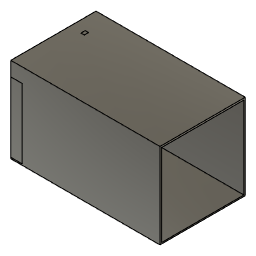
ufo-hanger-with-door (Autodesk Fusion 360 design; units mm, degrees)
Autodesk Fusion 360 part; units mm, degrees
sketch "Sketch1" plane through (0, 0, 0) normal (0, 1, 0) x (1, 0, 0)
  line L0 (0, -120) -> (101.6, -120)
  line L1 (101.6, -120) -> (101.6, 57.8)
  line L2 (101.6, 57.8) -> (0, 57.8)
  line L3 (0, 57.8) -> (0, -120)
  dimension "d1" = 101.6
  dimension "d2" = 177.8
  constraint horizontal L0
  constraint vertical L1
  constraint horizontal L2
  constraint vertical L3
  measures "d1" distance of L0.start L0.end
  measures "d2" distance of L0.start L2.end
extrude "Extrude1" add sketch "Sketch1" along normal blind 101.6 makes body 1
move_body "Move1" bodies 1 to x (0, 0, 1) y (0, 1, 0) z (-1, 0, 0) at (53.5039, 0, 53.5039)
sketch "Sketch2" plane through (-66.4961, 0, 0) normal (-1, 0, 0) x (0, -1, 0)
  line L0 (0, 53.5039) -> (0, 155.1039)
  line L1 (0, 155.1039) -> (-101.6, 155.1039)
  line L2 (-101.6, 155.1039) -> (-101.6, 53.5039)
  line L3 (-101.6, 53.5039) -> (0, 53.5039)
  line L4 (-100, 153) -> (-2, 153)
  line L5 (-2, 153) -> (-2, 55)
  line L6 (-2, 55) -> (-100, 55)
  line L7 (-100, 55) -> (-100, 153)
  constraint horizontal L4
  constraint vertical L5
  constraint horizontal L6
  constraint vertical L7
extrude "Extrude2" cut sketch "Sketch2" against normal blind 182 contours L4 L5 L6 L7 bodies 1
sketch "Sketch3" plane through (-66.4961, 0, 0) normal (-1, 0, 0) x (0, -1, 0)
  line L0 (-2, 153) -> (-2, 55)
  line L1 (-2, 55) -> (-100, 55)
  line L2 (-100, 55) -> (-100, 153)
  line L3 (-100, 153) -> (-2, 153)
  line L4 (0, 53.5039) -> (0, 155.1039)
  line L5 (0, 155.1039) -> (-101.6, 155.1039)
  line L6 (-101.6, 155.1039) -> (-101.6, 53.5039)
  line L7 (-101.6, 53.5039) -> (0, 53.5039)
  line L8 (-100, 153) -> (-2, 153)
  line L9 (-2, 153) -> (-2, 138)
  line L10 (-2, 138) -> (-100, 138)
  line L11 (-100, 138) -> (-100, 153)
  dimension "d7" = 15
  constraint horizontal L8
  constraint vertical L9
  constraint horizontal L10
  constraint vertical L11
  constraint coincident L2.end L3.start
  measures "d7" distance of L2.end L10.end
extrude "Extrude3" add sketch "Sketch3" against normal blind 2 contours L0 L2 L3 L8 L9 L10 L11 bodies 1
sketch "Sketch4" plane through (-66.4961, 0, 0) normal (-1, 0, 0) x (0, -1, 0)
  line L0 (-2, 138) -> (-2, 55)
  line L1 (-2, 55) -> (-100, 55)
  line L2 (-100, 55) -> (-100, 138)
  line L3 (-100, 138) -> (-2, 138)
  line L4 (0, 53.5039) -> (0, 155.1039)
  line L5 (0, 155.1039) -> (-101.6, 155.1039)
  line L6 (-101.6, 155.1039) -> (-101.6, 53.5039)
  line L7 (-101.6, 53.5039) -> (0, 53.5039)
  line L8 (-104, 138) -> (2, 138)
  line L9 (2, 138) -> (2, 55)
  line L10 (2, 55) -> (-104, 55)
  line L11 (-104, 55) -> (-104, 138)
  constraint horizontal L8
  constraint vertical L9
  constraint horizontal L10
  constraint vertical L11
extrude "Extrude4" cut sketch "Sketch4" against normal blind 13.5 contours L0 L4 L8 L10 | L0 L1 L2 L3 L8 L10 | L2 L6 L8 L10 | L4 L8 L9 L10 | L6 L8 L10 L11 bodies 1
sketch "Sketch5" plane through (0, 0, 155.1039) normal (0, 0, 1) x (-1, 0, 0)
  line L0 (66.4961, 0) -> (-111.3039, 0)
  line L1 (-111.3039, 0) -> (-111.3039, -101.6)
  line L2 (-111.3039, -101.6) -> (66.4961, -101.6)
  line L3 (66.4961, -101.6) -> (66.4961, 0)
  line L4 (60, -50) -> (56, -50)
  line L5 (56, -50) -> (56, -46)
  line L6 (56, -46) -> (60, -46)
  line L7 (60, -46) -> (60, -50)
  line L8 (60, -50) -> (56, -50)
  line L9 (56, -50) -> (33, -50)
  line L10 (33, -50) -> (33, -46)
  line L11 (33, -46) -> (56, -46)
  line L12 (56, -46) -> (56, -50)
  line L13 (33, -50) -> (29, -50)
  line L14 (29, -50) -> (29, -46)
  line L15 (29, -46) -> (33, -46)
  line L16 (33, -46) -> (33, -50)
  dimension "d12" = 4
  dimension "d13" = 4
  dimension "d14" = 4
  dimension "d15" = 23
  constraint horizontal L4
  constraint vertical L5
  constraint horizontal L6
  constraint vertical L7
  constraint horizontal L8
  constraint horizontal L9
  constraint vertical L10
  constraint horizontal L11
  constraint vertical L12
  constraint horizontal L13
  constraint vertical L14
  constraint horizontal L15
  constraint vertical L16
  measures "d12" distance of L4.start L4.end
  measures "d13" distance of L4.start L6.end
  measures "d14" distance of L4.end L4.start
  measures "d15" distance of L4.end L9.end
extrude "Extrude5" add sketch "Sketch5" against normal blind 14 separate body contours L4 L5 L6 L7 L8 L12 | L10 L13 L14 L15 L16 makes body 2 at (-57.3333, 46, 150.4372) makes body 3 at (-31.6667, 46, 145.7705)
sketch "Sketch6" plane through (-33, 0, 0) normal (-1, 0, 0) x (0, -1, 0)
  line L0 (-46, 155.1039) -> (-50, 155.1039)
  line L1 (-50, 155.1039) -> (-50, 141.1039)
  line L2 (-50, 141.1039) -> (-46, 141.1039)
  line L3 (-46, 141.1039) -> (-46, 155.1039)
  circle A0 centre (-48, 148) radius 0.7983
move_body "Move2" bodies 2 3 to x (1, 0, 0) y (0, 1, 0) z (0, 0, 1) at (-5, 0, 0)
sketch "Sketch7" plane through (0, 46, 0) normal (0, -1, 0) x (1, 0, 0)
  line L0 (-61, 155.1039) -> (-65, 155.1039)
  line L1 (-65, 155.1039) -> (-65, 141.1039)
  line L2 (-65, 141.1039) -> (-61, 141.1039)
  line L3 (-61, 141.1039) -> (-61, 155.1039)
  circle A0 centre (-62.9824, 148.1039) radius 0.6705
  circle A1 centre (-35.9824, 148.1039) radius 0.6705
extrude "Extrude7" cut sketch "Sketch7" against normal blind 9 contours A0 | A1 bodies 2 3
move_body "Move3" bodies 3 2 to x (1, 0, 0) y (0, 1, 0) z (0, 0, 1) at (0.5, 0, 0)
sketch "Sketch8" plane through (-66.4961, 0, 0) normal (-1, 0, 0) x (0, -1, 0)
  line L0 (-101.6, 138) -> (0, 138)
  line L1 (0, 138) -> (0, 155.1039)
  line L2 (0, 155.1039) -> (-101.6, 155.1039)
  line L3 (-101.6, 155.1039) -> (-101.6, 138)
  line L4 (-101.6, 138) -> (0, 138)
  line L5 (0, 138) -> (0, 55)
  line L6 (0, 55) -> (-101.6, 55)
  line L7 (-101.6, 55) -> (-101.6, 138)
  constraint horizontal L4
  constraint vertical L5
  constraint horizontal L6
  constraint vertical L7
  constraint coincident L0.start L3.end
extrude "Extrude8" add sketch "Sketch8" against normal blind 7 separate body contours L0 L4 L5 L6 L7 makes body 4
copy_body "Body->Comp1" bodies 4 removing the originals makes body 5 in component "Component"
combine "Combine1" operation add target body 1 tool bodies 2 3
copy_body "Body->Comp2" bodies 1 removing the originals makes body 6 in component "Component'"
sketch "Sketch9" plane through (0, 0, 155.1039) normal (0, 0, 1) x (-1, 0, 0)
  line L0 (66.4961, 0) -> (-111.3039, 0)
  line L1 (-111.3039, 0) -> (-111.3039, -101.6)
  line L2 (-111.3039, -101.6) -> (66.4961, -101.6)
  line L3 (66.4961, -101.6) -> (66.4961, 0)
  line L4 (52.869, -75) -> (48.8377, -75)
  line L5 (48.8377, -75) -> (48.8377, -70)
  line L6 (48.8377, -70) -> (52.869, -70)
  line L7 (52.869, -70) -> (52.869, -75)
  line L8 (66.4961, -69.9918) -> (52.7961, -69.9918)
  line L9 (52.7961, -69.9918) -> (52.7961, -75)
  line L10 (52.7961, -75) -> (66.4961, -75)
  line L11 (66.4961, -75) -> (66.4961, -69.9918)
  dimension "d26" = 13.7
  constraint horizontal L4
  constraint vertical L5
  constraint horizontal L6
  constraint vertical L7
  constraint horizontal L8
  constraint vertical L9
  constraint horizontal L10
  constraint vertical L11
  constraint coincident L3 L8.start
  measures "d26" distance of L8.start L8.end
extrude "Extrude9" add sketch "Sketch9" against normal blind 17 separate body contours L4 L5 L6 L9 makes body 7
copy_body "Body->Comp3" bodies 7 removing the originals makes body 8 in component "Component''"
extrude "Extrude1'" add 1 faces at (-59.4961, 67.7333, 110.3333) along direction (1, 0, 0) blind 6.5 on bodies 5 bodies 5 in component "Component"
component "Component" placed x (1, 0, 0) y (0, 1, 0) z (0, 0, 1) at (0, 0, 0)
component "Component'" placed x (1, 0, 0) y (0, 1, 0) z (0, 0, 1) at (0, 0, 0)
component "Component''" placed x (1, 0, 0) y (0, 1, 0) z (0, 0, 1) at (0, 0, 0)
